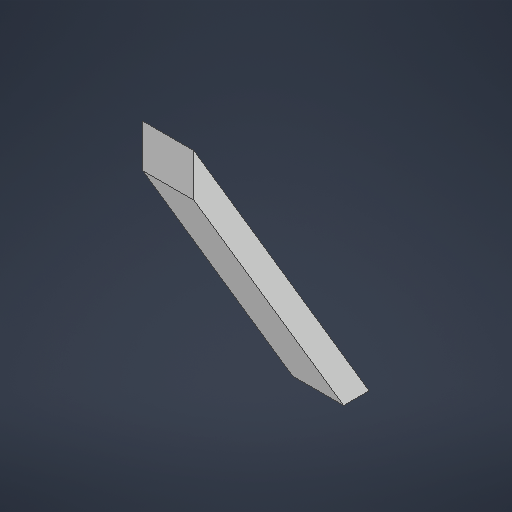
# Autodesk Inventor part: S_2x4x31.38
Saved by Autodesk Inventor 2027.1 (Build 311270010, 270A)
## iProperties
Created: 2026-09-01
Part Number: S_2x4x31.38
Material: Generic
Document SubType Name: Modeling
Designer: jorda
Density: 1 g/cm^3
Appearance: Default
Author: jorda
Autodesk Inventor part; units mm, degrees
ref_plane "YZ Plane" through (0, 0, 0) normal (1, 0, 0) x (0, 1, 0)
ref_plane "XZ Plane" through (0, 0, 0) normal (0, 1, 0) x (-1, 0, 0)
ref_plane "XY Plane" through (0, 0, 0) normal (0, 0, 1) x (1, 0, 0)
sketch "Sketch1" plane through (0, 0, 0) normal (1, 0, 0) x (0, 1, 0)
  line L0 (0, -406.4) -> (0, -362.1127)
  line L1 (431.3757, -106.4826) -> (439.6152, -101.6)
  line L2 (431.3757, -106.4826) -> (0, -362.1127)
  line L3 (0, -406.4) -> (0, -362.1127)
  line L4 (0, -406.4) -> (0, -362.1127)
  line L5 (514.35, -101.6) -> (0, -406.4)
  line L6 (439.6152, -101.6) -> (514.35, -101.6)
  point P0 (0, 0)
  point P1 (0, -362.1127)
  point P2 (0, -362.1127)
  constraints: 14 end point, 1 perpendicular, 1 vertical
extrude "Extrusion1" add sketch "Sketch1" along normal blind 88.9
body "Solid1"
